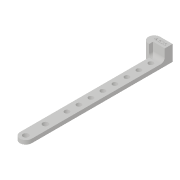
# Autodesk Inventor part: CollectorArmRear4_525long
Saved by Autodesk Inventor 2018 (Build 220112000, 112)
## iProperties
Created: 2019-02-19
Part Number: CollectorArmRear4_525long
Material: Generic
Document SubType Name: Modeling
Designer: ball
Density: 1 g/cm^3
Appearance: Default
Author: ball
Autodesk Inventor part; units mm, degrees
note: some values were not read from the file. Chosen so that the rebuilt part matches the saved one: direction of "Emboss1".
ref_plane "YZ Plane" through (0, 0, 0) normal (1, 0, 0) x (0, 1, 0)
ref_plane "XZ Plane" through (0, 0, 0) normal (0, 1, 0) x (-1, 0, 0)
ref_plane "XY Plane" through (0, 0, 0) normal (0, 0, 1) x (1, 0, 0)
sketch "Sketch1" plane through (0, 0, 0) normal (0, 1, 0) x (-1, 0, 0)
  line L0 (0, 0) -> (10.16, 0)
  line L1 (9.525, 9.6012) -> (9.525, 114.935)
  line L2 (0, 114.935) -> (0, 0)
  circle A0 centre (4.7625, 114.935) radius 2.2479
  circle A1 centre (4.7625, 98.933) radius 2.2479
  circle A2 centre (4.7625, 81.3816) radius 1.9685
  arc A3 (10.16, 0) -> (10.16, 9.6012) centre (10.16, 4.8006) ccw
  line L3 (10.16, 9.6012) -> (9.525, 9.6012)
  circle A4 centre (4.7625, 71.6026) radius 1.9685
  circle A5 centre (4.7625, 61.8236) radius 1.9685
  circle A6 centre (4.7625, 52.0446) radius 1.9685
  circle A7 centre (4.7625, 42.2656) radius 1.9685
  circle A8 centre (4.7625, 32.4866) radius 1.9685
  circle A9 centre (4.7625, 22.7076) radius 1.9685
  circle A10 centre (4.7625, 12.9286) radius 1.9685
  arc A11 (9.525, 114.935) -> (0, 114.935) centre (4.7625, 114.9855) ccw
  dimension "d0" = 9.525
  dimension "d4" = 4.4958
  dimension "d5" = 4.4958
  dimension "d6" = 16.002
  dimension "d7" = 3.937
  dimension "d8" = 17.5514
  dimension "d16" = 4.8006
  dimension "d17" = 10.16
  dimension "d18" = 114.935
  dimension "d21" = 9.779
  dimension "d27" = 4.7628
  dimension "d28" = 0
  dimension "d29" = 0
  constraints: 12 centre point, 8 end point, 4 point on circle, 2 perpendicular, 1 coincident, 1 horizontal, 1 parallel, 1 vertical, 14 other
  measures "d0" distance of L2.start L1.end
  measures "d4" diameter of A0
  measures "d5" diameter of A1
  measures "d6" distance of A1.centre A0.centre
  measures "d7" diameter of A2
  measures "d8" distance of A2.centre A1.centre
  measures "d16" distance from line of L0 point (10.16, 4.801)
  measures "d17" distance from line of L2 point (10.16, 4.801)
  measures "d18" distance from line of L0 A0.centre
  measures "d21" distance of A2.centre A4.centre
  measures "d27" radius of A11
  measures "d28" vertical distance of L1.end A0.centre
  measures "d29" vertical distance of L2.start A0.centre
extrude "Extrusion1" add sketch "Sketch1" along normal blind 3.175
sketch "Sketch2" plane through (0, 3.175, 0) normal (0, 1, 0) x (1, 0, 0)
  line L0 (-9.525, -9.6012) -> (-9.525, -6.35)
  line L1 (-9.525, -6.35) -> (0, -6.35)
  line L2 (0, -114.935) -> (0, 0) projected
  line L3 (0, -6.35) -> (0, 0)
  arc A0 (-10.16, 0) -> (-10.16, -9.6012) centre (-10.16, -4.8006) ccw projected
  arc A1 (-10.16, 0) -> (-10.239, -9.6012) centre (-10.1597, -4.8009) ccw
  line L4 (-10.16, -9.6012) -> (-9.525, -9.6012) projected
  line L5 (-9.525, -9.6012) -> (-10.16, -9.6012)
  line L6 (0, 0) -> (-10.16, 0) projected
  line L7 (-10.16, 0) -> (0, 0)
  constraints: 10 end point, 3 point on circle, 2 perpendicular, 1 centre point, 1 collinear, 1 horizontal, 1 vertical
extrude "Extrusion2" add sketch "Sketch2" along normal blind 9.525
fillet "Fillet1" radius 3.175 2 edges at (-4.7625, 3.175, 6.35) (-9.525, 3.175, 7.9756)
sketch "Sketch5" plane through (0, 12.7, 0) normal (0, 1, 0) x (1, 0, 0)
  line L0 (-11.1912, 0.0281) -> (-1.5184, 0.0281) construction
  line L1 (-1.5184, 0.0281) -> (-1.5184, -6.3829) construction
  line L2 (-1.5184, -6.3829) -> (-11.1912, -6.3829) construction
  line L3 (-11.1912, -6.3829) -> (-11.1912, 0.0281) construction
  line L4 (-9.1953, -3.8525) -> (-9.5391, -3.8525)
  line L5 (-9.5391, -3.8525) -> (-9.5391, -4.4515)
  line L6 (-9.5391, -4.4515) -> (-10.1545, -4.4515)
  line L7 (-10.1545, -4.4515) -> (-10.1545, -3.8525)
  line L8 (-10.1545, -3.8525) -> (-11.2742, -3.8525)
  line L9 (-11.2742, -3.8525) -> (-11.2742, -3.3791)
  line L10 (-11.2742, -3.3791) -> (-10.1751, -1.9053)
  line L11 (-10.1751, -1.9053) -> (-9.5391, -1.9053)
  line L12 (-9.5391, -1.9053) -> (-9.5391, -3.3956)
  line L13 (-9.5391, -3.3956) -> (-9.1953, -3.3956)
  line L14 (-9.1953, -3.3956) -> (-9.1953, -3.8525)
  line L15 (-10.1545, -3.3956) -> (-10.1545, -2.5311)
  line L16 (-10.1545, -2.5311) -> (-10.7988, -3.3956)
  line L17 (-10.7988, -3.3956) -> (-10.1545, -3.3956)
  line L18 (-8.2793, -4.4453) -> (-8.8824, -4.4453)
  line L19 (-8.8824, -4.4453) -> (-8.8824, -3.7743)
  line L20 (-8.8824, -3.7743) -> (-8.2793, -3.7743)
  line L21 (-8.2793, -3.7743) -> (-8.2793, -4.4453)
  spline S0 degree 2 poles (-5.9678, -3.5849) (-5.9678, -3.7846) (-6.1037, -4.1222) (-6.2375, -4.2436) knots 0 0 0 1 2 2 2
  spline S1 degree 2 poles (-6.2375, -4.2436) (-6.3713, -4.3651) (-6.7376, -4.4989) (-7.0052, -4.4989) knots 0 0 0 1 2 2 2
  spline S2 degree 2 poles (-7.0052, -4.4989) (-7.2893, -4.4968) (-7.6968, -4.4042) (-7.8306, -4.3445) knots 0 0 0 1 2 2 2
  line L22 (-7.8306, -4.3445) -> (-7.8306, -3.7908)
  line L23 (-7.8306, -3.7908) -> (-7.773, -3.7908)
  spline S3 degree 2 poles (-7.773, -3.7908) (-7.7236, -3.8175) (-7.6042, -3.8875) (-7.5075, -3.9246) knots 0 0 0 1 2 2 2
  spline S4 degree 2 poles (-7.5075, -3.9246) (-7.4169, -3.9596) (-7.2296, -4.0069) (-7.1164, -4.0069) knots 0 0 0 1 2 2 2
  spline S5 degree 2 poles (-7.1164, -4.0069) (-7.0176, -4.0069) (-6.787, -3.9575) (-6.7171, -3.8916) knots 0 0 0 1 2 2 2
  spline S6 degree 2 poles (-6.7171, -3.8916) (-6.6656, -3.8402) (-6.608, -3.7146) (-6.608, -3.6096) knots 0 0 0 1 2 2 2
  spline S7 degree 2 poles (-6.608, -3.6096) (-6.608, -3.5191) (-6.6821, -3.3915) (-6.7418, -3.3524) knots 0 0 0 1 2 2 2
  spline S8 degree 2 poles (-6.7418, -3.3524) (-6.8282, -3.2947) (-7.0752, -3.2618) (-7.1637, -3.2618) knots 0 0 0 1 2 2 2
  spline S9 degree 2 poles (-7.1637, -3.2618) (-7.3037, -3.2618) (-7.5692, -3.3071) (-7.666, -3.3318) knots 0 0 0 1 2 2 2
  line L24 (-7.666, -3.3318) -> (-7.7215, -3.3318)
  line L25 (-7.7215, -3.3318) -> (-7.7215, -1.9053)
  line L26 (-7.7215, -1.9053) -> (-6.0378, -1.9053)
  line L27 (-6.0378, -1.9053) -> (-6.0378, -2.3849)
  line L28 (-6.0378, -2.3849) -> (-7.1184, -2.3849)
  line L29 (-7.1184, -2.3849) -> (-7.1184, -2.8069)
  spline S10 degree 2 poles (-7.1184, -2.8069) (-7.067, -2.8028) (-6.925, -2.7987) (-6.8858, -2.7987) knots 0 0 0 1 2 2 2
  spline S11 degree 2 poles (-6.8858, -2.7987) (-6.7027, -2.7987) (-6.3939, -2.8728) (-6.2725, -2.9489) knots 0 0 0 1 2 2 2
  spline S12 degree 2 poles (-6.2725, -2.9489) (-6.1284, -3.0436) (-5.9678, -3.3585) (-5.9678, -3.5849) knots 0 0 0 1 2 2 2
  line L30 (-3.6851, -4.4453) -> (-5.552, -4.4453)
  line L31 (-5.552, -4.4453) -> (-5.552, -4.0316)
  spline S13 degree 2 poles (-5.552, -4.0316) (-5.3153, -3.8422) (-4.9366, -3.5088) (-4.7946, -3.3585) knots 0 0 0 1 2 2 2
  spline S14 degree 2 poles (-4.7946, -3.3585) (-4.6073, -3.163) (-4.4405, -2.8645) (-4.4405, -2.7081) knots 0 0 0 1 2 2 2
  spline S15 degree 2 poles (-4.4405, -2.7081) (-4.4405, -2.5311) (-4.6525, -2.3417) (-4.8419, -2.3417) knots 0 0 0 1 2 2 2
  spline S16 degree 2 poles (-4.8419, -2.3417) (-4.9387, -2.3417) (-5.1116, -2.3891) (-5.2001, -2.4261) knots 0 0 0 1 2 2 2
  spline S17 degree 2 poles (-5.2001, -2.4261) (-5.2865, -2.4652) (-5.41, -2.5475) (-5.4409, -2.5681) knots 0 0 0 1 2 2 2
  line L32 (-5.4409, -2.5681) -> (-5.4903, -2.5681)
  line L33 (-5.4903, -2.5681) -> (-5.4903, -2.0144)
  spline S18 degree 2 poles (-5.4903, -2.0144) (-5.3833, -1.963) (-4.9263, -1.8559) (-4.7143, -1.8559) knots 0 0 0 1 2 2 2
  spline S19 degree 2 poles (-4.7143, -1.8559) (-4.2615, -1.8559) (-3.7963, -2.2594) (-3.7963, -2.6237) knots 0 0 0 1 2 2 2
  spline S20 degree 2 poles (-3.7963, -2.6237) (-3.7963, -2.8481) (-4.0083, -3.2803) (-4.2532, -3.5273) knots 0 0 0 1 2 2 2
  spline S21 degree 2 poles (-4.2532, -3.5273) (-4.4076, -3.6796) (-4.6978, -3.9163) (-4.7616, -3.9657) knots 0 0 0 1 2 2 2
  line L34 (-4.7616, -3.9657) -> (-3.6851, -3.9657)
  line L35 (-3.6851, -3.9657) -> (-3.6851, -4.4453)
  spline S22 degree 2 poles (-1.5177, -3.5849) (-1.5177, -3.7846) (-1.6535, -4.1222) (-1.7873, -4.2436) knots 0 0 0 1 2 2 2
  spline S23 degree 2 poles (-1.7873, -4.2436) (-1.9211, -4.3651) (-2.2875, -4.4989) (-2.5551, -4.4989) knots 0 0 0 1 2 2 2
  spline S24 degree 2 poles (-2.5551, -4.4989) (-2.8391, -4.4968) (-3.2467, -4.4042) (-3.3805, -4.3445) knots 0 0 0 1 2 2 2
  line L36 (-3.3805, -4.3445) -> (-3.3805, -3.7908)
  line L37 (-3.3805, -3.7908) -> (-3.3228, -3.7908)
  spline S25 degree 2 poles (-3.3228, -3.7908) (-3.2734, -3.8175) (-3.1541, -3.8875) (-3.0573, -3.9246) knots 0 0 0 1 2 2 2
  spline S26 degree 2 poles (-3.0573, -3.9246) (-2.9668, -3.9596) (-2.7794, -4.0069) (-2.6662, -4.0069) knots 0 0 0 1 2 2 2
  spline S27 degree 2 poles (-2.6662, -4.0069) (-2.5674, -4.0069) (-2.3369, -3.9575) (-2.2669, -3.8916) knots 0 0 0 1 2 2 2
  spline S28 degree 2 poles (-2.2669, -3.8916) (-2.2155, -3.8402) (-2.1578, -3.7146) (-2.1578, -3.6096) knots 0 0 0 1 2 2 2
  spline S29 degree 2 poles (-2.1578, -3.6096) (-2.1578, -3.5191) (-2.2319, -3.3915) (-2.2916, -3.3524) knots 0 0 0 1 2 2 2
  spline S30 degree 2 poles (-2.2916, -3.3524) (-2.3781, -3.2947) (-2.6251, -3.2618) (-2.7136, -3.2618) knots 0 0 0 1 2 2 2
  spline S31 degree 2 poles (-2.7136, -3.2618) (-2.8535, -3.2618) (-3.1191, -3.3071) (-3.2158, -3.3318) knots 0 0 0 1 2 2 2
  line L38 (-3.2158, -3.3318) -> (-3.2714, -3.3318)
  line L39 (-3.2714, -3.3318) -> (-3.2714, -1.9053)
  line L40 (-3.2714, -1.9053) -> (-1.5877, -1.9053)
  line L41 (-1.5877, -1.9053) -> (-1.5877, -2.3849)
  line L42 (-1.5877, -2.3849) -> (-2.6683, -2.3849)
  line L43 (-2.6683, -2.3849) -> (-2.6683, -2.8069)
  spline S32 degree 2 poles (-2.6683, -2.8069) (-2.6168, -2.8028) (-2.4748, -2.7987) (-2.4357, -2.7987) knots 0 0 0 1 2 2 2
  spline S33 degree 2 poles (-2.4357, -2.7987) (-2.2525, -2.7987) (-1.9438, -2.8728) (-1.8223, -2.9489) knots 0 0 0 1 2 2 2
  spline S34 degree 2 poles (-1.8223, -2.9489) (-1.6782, -3.0436) (-1.5177, -3.3585) (-1.5177, -3.5849) knots 0 0 0 1 2 2 2
  point P0 (0, 0)
  constraints: 2 other
emboss "Emboss1" sketch "Sketch5" operation cut depth 0.762 direction (0, -1, 0)
body "Solid1"
